4mm (Autodesk Fusion 360 design; units mm, degrees)
Autodesk Fusion 360 part; units mm, degrees
sketch "Sketch1" plane through (0, 0, 0) normal (0, 1, 0) x (1, 0, 0)
  line L0 (0, 0) -> (0, -1.8)
  line L1 (0, -1.8) -> (0.1, -1.9)
  line L2 (0.1, -1.9) -> (0.5, -1.9)
  line L3 (0.5, -1.9) -> (0.5, 0)
  line L4 (0.5, 0) -> (0, 0)
  line L5 (0, -1.505) -> (-0.25, -1.505)
  line L6 (-0.25, -1.505) -> (-0.25, -1.4)
  line L7 (-0.25, -1.4) -> (-0.75, -1.4)
  line L8 (-0.75, -1.4) -> (-0.75, -1.505)
  line L9 (-0.75, -1.505) -> (-1.9, -1.505)
  line L10 (-1.9, -1.505) -> (-2.3, -1.3978)
  line L11 (-2.3, -1.3978) -> (-2.3, -1)
  line L12 (-2.3, -1) -> (0, -1)
  dimension "d2" = 0.1
  dimension "d3" = 0.1
  dimension "d5" = 1
  dimension "d6" = 1.4
  dimension "d7" = 0.25
  dimension "d8" = 0.5
  dimension "d10" = 0.4
  dimension "d11" = 0.1072
  dimension "d12" = 2.3
  dimension "d27" = 1.9
  dimension "d28" = 1.505
  dimension "d29" = 0.5
  constraint coincident L0.start L4.end
  constraint vertical L0
  constraint perpendicular L0 L2
  constraint perpendicular L2 L3
  constraint perpendicular L0 L4
  constraint coincident L0 L5.start
  constraint perpendicular L0 L5
  constraint perpendicular L5 L6
  constraint perpendicular L0 L7
  constraint perpendicular L7 L8
  constraint perpendicular L8 L9
  constraint perpendicular L9 L11
  constraint perpendicular L8 L12
  constraint collinear L5 L9
  measures "d2" horizontal distance of L0.end L1.end
  measures "d3" vertical distance of L0.end L1.end
  measures "d5" distance of L0.start L12
  measures "d6" distance of L0.start L7
  measures "d7" distance of L5.start L5.end
  measures "d8" distance of L6.end L7.end
  measures "d10" horizontal distance of L9.end L10.end
  measures "d11" vertical distance of L9.end L10.end
  measures "d12" distance of L0 L11
  measures "d27" distance of L2 L4
  measures "d28" distance of L0.start L9
  measures "d29" distance of L0 L3
revolve "Revolve1" add sketch "Sketch1" angle 360 about axis through (0.5, 0, 0) along (-1, 0, 0)
sketch "Sketch3" plane through (0.5, 0, 0) normal (1, 0, 0) x (0, 1, 0)
  circle A0 centre (0, 0) radius 1.9
  arc A1 (-1.1535, -1.4785) -> (-0.8923, -1.5532) centre (-0.9293, -1.1884) ccw
  line L0 (-1.7528, 0.3686) -> (-1.6405, 0.1157)
  arc A2 (0.998, -0.096) -> (1.8427, 0.3471) centre (1.4581, 0.0535) cw
  line L1 (-0.1911, 1.7806) -> (-0.3968, 1.5956)
  arc A3 (-1.6405, 0.1157) -> (-1.5225, -0.0306) centre (-1.3109, 0.2606) ccw
  arc A4 (0.0642, 1.8737) -> (-0.1911, 1.7806) centre (0.0532, 1.5071) ccw
  arc A5 (1.8427, 0.3471) -> (1.8022, 0.5176) centre (0.0001, -0.0005) ccw
  arc A6 (-0.7512, 0.6639) -> (-1.6951, 0.8019) centre (-1.2114, 0.8135) cw
  line L2 (1.2138, 0.9192) -> (0.3996, 0.9193)
  line L3 (1.2012, -1.3288) -> (1.259, -1.0582)
  arc A7 (-1.6951, 0.8019) -> (-1.7625, 0.6402) centre (0, 0.0001) ccw
  arc A8 (-1.7625, 0.6402) -> (-1.7528, 0.3686) centre (-1.4173, 0.5165) ccw
  line L4 (-0.4414, -1.4576) -> (0.2173, -0.979)
  arc A9 (1.259, -1.0582) -> (1.2496, -0.8705) centre (0.9071, -0.9817) ccw
  arc A10 (-0.8637, -0.5094) -> (-1.2865, -1.3644) centre (-1.148, -0.9008) cw
  arc A11 (1.0495, -1.5542) -> (1.2012, -1.3288) centre (0.8428, -1.2512) ccw
  arc A12 (1.3952, 0.8701) -> (1.2138, 0.9192) centre (1.2137, 0.5592) ccw
  arc A13 (0.8998, -1.6454) -> (1.0495, -1.5542) centre (-0.0002, -0.0004) ccw
  arc A14 (-1.2865, -1.3644) -> (-1.1535, -1.4785) centre (-0.0001, -0.0001) ccw
  arc A15 (1.8022, 0.5176) -> (1.6347, 0.7316) centre (1.4502, 0.4147) ccw
  arc A16 (0.3996, 0.9193) -> (0.2389, 1.8595) centre (0.3993, 1.4031) cw
  line L5 (1.2496, -0.8705) -> (0.998, -0.096)
  arc A17 (-0.3968, 1.5956) -> (-0.4996, 1.4382) centre (-0.1572, 1.3269) ccw
  line L6 (-0.8923, -1.5532) -> (-0.6171, -1.5245)
  line L7 (1.6347, 0.7316) -> (1.3952, 0.8701)
  line L8 (-1.5225, -0.0306) -> (-0.8637, -0.5094)
  arc A18 (0.2173, -0.979) -> (0.8998, -1.6454) centre (0.5017, -1.3705) cw
  line L9 (-0.4996, 1.4382) -> (-0.7512, 0.6639)
  arc A19 (-0.6171, -1.5245) -> (-0.4414, -1.4576) centre (-0.653, -1.1663) ccw
  arc A20 (0.2389, 1.8595) -> (0.0642, 1.8737) centre (0, -0.0003) ccw
  circle A21 centre (0, 0) radius 1.8748
  constraint coincident A0.centre A21.centre
  constraint coincident A16.end A21
extrude "Extrude2" add sketch "Sketch3" along normal blind 1.46 contours A1 L0 A2 L1 A3 A4 A5 A6 L2 L3 A7 A8 L4 A9 A10 A11 A12 A13 A14 A15 A16 L5 A17 L6 L7 L8 A18 L9 A19 A20 A21
move_body "Move1" bodies 1 to x (0, 0, 1) y (0, 1, 0) z (-1, 0, 0) at (-4.25, 0, 0.35)
equation "d5 = ( 2 / 2 ) * 1 mm"
equation "d6 = ( 2.8 / 2 ) * 1 mm"
equation "d25 = 1.960 mm - 0.5 mm"
equation "d27 = 3.8 mm / 2"
equation "d28 = var / 2"
equation "var = 3.010 mm"
